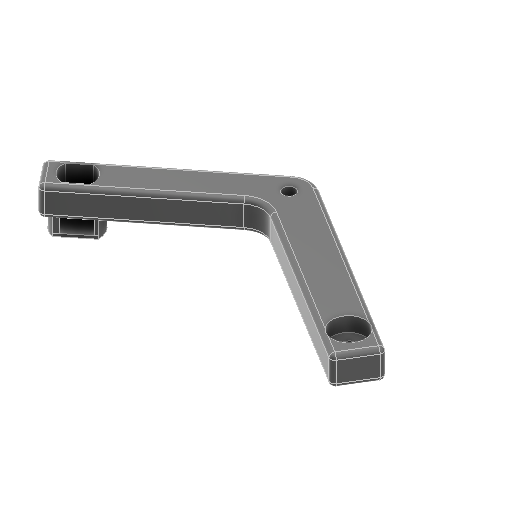
# Autodesk Inventor part: bogie
Saved by Autodesk Inventor 2025 (Build 290162010, 162A)
## iProperties
Created: 2024-08-06
Part Number: bogie
Material: Generic
Document SubType Name: Modeling
Designer: Pauline Simonnet
Density: 1 g/cm^3
Appearance: Smooth - Black
Author: Pauline Simonnet
Autodesk Inventor part; units mm, degrees
ref_plane "YZ Plane" through (0, 0, 0) normal (1, 0, 0) x (0, 1, 0)
ref_plane "XZ Plane" through (0, 0, 0) normal (0, 1, 0) x (-1, 0, 0)
ref_plane "XY Plane" through (0, 0, 0) normal (0, 0, 1) x (1, 0, 0)
sketch "Sketch1" plane through (0, 0, 0) normal (0, 1, 0) x (-1, 0, 0)
  line L0 (-461.117288, -185.63027) -> (-373.951633, -116.199404)
  line L1 (-373.951633, -116.199404) -> (-461.117288, -185.63027)
  line L2 (-461.117288, -185.63027) -> (-576.400041, -115.091965)
  line L3 (-576.400041, -115.091965) -> (-591.013873, -138.975765)
  line L4 (-591.013873, -138.975765) -> (-462.638447, -217.525112)
  line L5 (-373.951633, -116.199404) -> (-358.998599, -134.971905)
  line L6 (-358.998599, -134.971905) -> (-462.638447, -217.525112)
  line L7 (-462.638447, -217.525112) -> (-451.010555, -198.521319) construction
  line L8 (-462.638447, -217.525112) -> (-476.037837, -200.703103) construction
  circle A0 centre (-463.768354, -199.253824) radius 4.2
  circle A1 centre (-566.6471, -137.472317) radius 4.3
  line L9 (-369.889547, -139.044495) -> (-380.752312, -147.697115)
  line L10 (-379.951692, -126.412167) -> (-390.814458, -135.064786)
  line L11 (-375.32093, -143.370805) -> (-385.383075, -130.738476) construction
  line L12 (-366.475116, -125.585654) -> (-380.352002, -137.054641) construction
  arc A2 (-369.889547, -139.044495) -> (-379.951692, -126.412167) centre (-380.352002, -137.054641) ccw
  arc A3 (-390.814458, -135.064786) -> (-380.752312, -147.697115) centre (-380.352002, -137.054641) ccw
  point P0 (0, 0)
  dimension "d17" = 110
  dimension "d18" = 28
  dimension "d19" = 24
  dimension "d20" = 90
  dimension "d21" = 90
  dimension "d23" = 8.6
  dimension "d24" = 8.4
  dimension "d25" = 20
  dimension "d26" = 14
  dimension "d29" = 10.5
  dimension "d30" = 10.5
  dimension "d31" = 140
  dimension "d32" = 122
  dimension "d43" = 16.15
  dimension "d46" = 10.65
  dimension "d47" = 18
  constraints: 26 end point, 4 centre point, 4 midpoint, 4 point on circle, 1 coincident, 1 collinear, 1 perpendicular
  measures "d17" angle of L2 L0
  measures "d18" distance between parallel lines of L4 L2
  measures "d19" distance between parallel lines of L0 L6
  measures "d20" angle of L8 L6
  measures "d21" angle of L4 L7
  measures "d23" diameter of A1
  measures "d24" diameter of A0
  measures "d25" distance from line of L3 A1.centre
  measures "d26" distance from line of A1.centre L2
  measures "d29" distance from line of A0.centre L7
  measures "d30" distance from line of L8 A0.centre
  measures "d31" distance from line of L3 A0.centre
  measures "d32" distance from line of A0.centre L5
  measures "d43" distance between parallel lines of L10 L9
  measures "d46" radius of A3
  measures "d47" distance between parallel lines of L11 L5
extrude "Extrusion1" add sketch "Sketch1" along normal blind 20
fillet "Fillet1" radius 15 1 edges at (461.1173, 10, -185.6303)
fillet "Fillet2" radius 15 1 edges at (462.6384, 10, -217.5251)
fillet "Fillet3" radius 3 3 edges at (461.3217, 20, -182.325) (523.2382, 20, -147.6202) (413.4268, 20, -147.6429)
fillet "Fillet4" radius 3 3 edges at (462.8428, 20, -214.2198) (531.3057, 20, -175.5095) (406.7108, 20, -172.9766)
fillet "Fillet5" radius 3 3 edges at (462.8428, 0, -214.2198) (531.3057, 0, -175.5095) (406.7108, 0, -172.9766)
fillet "Fillet6" radius 3 3 edges at (461.3217, 0, -182.325) (523.2382, 0, -147.6202) (413.4268, 0, -147.6429)
fillet "Fillet7" radius 3 8 edges at (590.5553, 19.1213, -138.2263) (583.707, 20, -127.0339) (576.8586, 19.1213, -115.8415) (576.4, 10, -115.092) (576.8586, 0.8787, -115.8415) (583.707, 0, -127.0339) (590.5553, 0.8787, -138.2263) (591.0139, 10, -138.9758)
fillet "Fillet8" radius 3 8 edges at (373.4042, 0.8787, -116.8867) (373.9516, 10, -116.1994) (373.4042, 19.1213, -116.8867) (366.4751, 20, -125.5857) (359.5461, 19.1213, -134.2846) (358.9986, 10, -134.9719) (359.5461, 0.8787, -134.2846) (366.4751, 0, -125.5857)
sketch "Sketch4" plane through (0, 0, 0) normal (0, -1, 0) x (1, 0, 0)
  arc A0 (379.951692, -126.412167) -> (369.889547, -139.044495) centre (380.352002, -137.054641) ccw
  line L0 (368.362548, -139.106647) -> (381.790516, -149.80255)
  line L1 (369.889547, -139.044495) -> (380.752312, -147.697115)
  line L2 (365.950797, -139.742524) -> (380.584185, -151.398592)
  line L3 (394.697833, -137.054641) -> (377.324066, -122.721077)
  line L4 (451.032754, -181.432941) -> (374.429066, -120.415096)
  arc A1 (377.324066, -122.721077) -> (365.950797, -139.742524) centre (380.352002, -137.054641) ccw
  arc A2 (380.584185, -151.398592) -> (394.689059, -136.552975) centre (380.352002, -137.054641) ccw
  arc A3 (380.052693, -124.894536) -> (368.362548, -139.106647) centre (380.352002, -137.054641) ccw
  arc A4 (381.790516, -149.80255) -> (393.053252, -135.249991) centre (380.352002, -137.054641) ccw
  point P0 (0, 0)
  point P1 (379.961653, -124.897118)
  point P2 (393.114108, -135.748048)
  dimension "d60" = 0
  dimension "d61" = 0
  dimension "d64" = 1
  dimension "d65" = 2
  constraints: 9 point on circle, 6 end point, 4 centre point, 4 point on line, 1 coincident, 1 parallel
  measures "d60" distance of A0.centre A3.centre
  measures "d61" distance of A0.centre A3.centre
  measures "d64" distance between parallel lines of L1 L0
  measures "d65" distance between parallel lines of L0 L2
extrude "Extrusion4" add sketch "Sketch4" along normal blind 10 contours L0 A4 L3 A2 L2 A1 A3
sketch "Sketch5" plane through (0, -10, 0) normal (0, -1, 0) x (1, 0, 0)
  arc A0 (383.884165, -150.958837) -> (394.697833, -137.054641) centre (380.352002, -137.054641) ccw
  line L0 (394.697833, -137.054641) -> (377.413043, -123.131119)
  arc A1 (380.584185, -151.398592) -> (394.697833, -137.054641) centre (380.352002, -137.054641) ccw
  line L1 (380.584185, -151.398592) -> (365.950797, -139.742524)
  line L2 (365.950797, -139.742524) -> (380.584185, -151.398592)
  arc A2 (380.584185, -151.398592) -> (394.696971, -136.897401) centre (380.352002, -137.054641) ccw
  arc A3 (377.232481, -122.74073) -> (365.950797, -139.742524) centre (380.352002, -137.054641) ccw
  line L3 (394.696971, -136.897401) -> (377.232481, -122.74073)
  point P0 (0, 0)
  point P1 (377.520119, -122.877245)
  constraints: 8 end point, 4 point on circle, 2 centre point, 1 coincident
extrude "Extrusion5" add sketch "Sketch5" along normal blind 2
sketch "Sketch6" plane through (0, 0, 0) normal (0, -1, 0) x (1, 0, 0)
  circle A0 centre (463.768354, -199.253824) radius 11.425
  circle A1 centre (463.768354, -199.253824) radius 4.2
  point P0 (0, 0)
  dimension "d70" = 0
  dimension "d71" = 0
  dimension "d72" = 22.85
  constraints: 1 centre point
  measures "d70" distance of A1.centre A0.centre
  measures "d71" distance of A1.centre A0.centre
  measures "d72" diameter of A0
extrude "Extrusion6" cut sketch "Sketch6" against normal blind 10
sketch "Schizzo8" plane through (0, 20, 0) normal (0, 1, 0) x (1, 0, 0)
  circle A0 centre (566.6471, 137.472317) radius 4.3
  circle A1 centre (566.6471, 137.472317) radius 11.425
  point P0 (0, 0)
  dimension "d77" = 22.85
  constraints: 1 centre point, 1 coincident
  measures "d77" diameter of A1
extrude "Estrusione8" cut sketch "Schizzo8" against normal blind 10 contours A0 | A1
body "Solid1"
